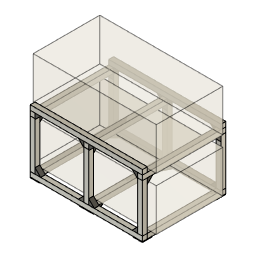
Battery Rack v4 (Autodesk Fusion 360 design; units mm, degrees)
Autodesk Fusion 360 part; units mm, degrees
note: some values were not read from the file. Chosen so that the rebuilt part matches the saved one: which bodies a step acts on.
sketch "Sketch1" plane through (0, 0, 0) normal (0, 0, 1) x (1, 0, 0)
  line L0 (-350, 260) -> (350, 260)
  line L1 (350, 260) -> (350, 230)
  line L2 (350, 230) -> (-350, 230)
  line L3 (-350, 230) -> (-350, 260)
  line L4 (-350, 230) -> (-320, 230)
  line L5 (-320, 230) -> (-320, -230)
  line L6 (-320, -230) -> (-350, -230)
  line L7 (-350, -230) -> (-350, 230)
  line L8 (-350, -230) -> (350, -230)
  line L9 (350, -230) -> (350, -260)
  line L10 (350, -260) -> (-350, -260)
  line L11 (-350, -260) -> (-350, -230)
  line L12 (350, -230) -> (320, -230)
  line L13 (320, -230) -> (320, 230)
  line L14 (320, 230) -> (350, 230)
  line L15 (350, 230) -> (350, -230)
  line L16 (0, 260) -> (0, -260) construction
  line L17 (-15, 230) -> (15, 230)
  line L18 (15, 230) -> (15, -230)
  line L19 (15, -230) -> (-15, -230)
  line L20 (-15, -230) -> (-15, 230)
  line L21 (350, 0) -> (-350, 0) construction
  line L22 (0, 1.75) -> (0, 22.5)
  line L23 (1.75, 0) -> (22.5, 0)
  dimension "d1" = 700
  dimension "d2" = 30
  dimension "d3" = 30
  dimension "d6" = 30
  dimension "d7" = 30
  dimension "d9" = 30
  dimension "d11" = 15
  dimension "d70" = 460
  constraint horizontal L0
  constraint vertical L1
  constraint horizontal L2
  constraint vertical L3
  constraint horizontal L4
  constraint vertical L5
  constraint horizontal L6
  constraint vertical L7
  constraint horizontal L8
  constraint vertical L9
  constraint horizontal L10
  constraint vertical L11
  constraint horizontal L12
  constraint vertical L13
  constraint horizontal L14
  constraint vertical L15
  constraint midpoint L0 L16.start
  constraint midpoint L10 L16.end
  constraint horizontal L17
  constraint vertical L18
  constraint horizontal L19
  constraint vertical L20
  constraint coincident L2 L17.start
  constraint midpoint L15 L21.start
  constraint midpoint L7 L21.end
  constraint collinear L16 L22
  constraint collinear L21 L23
  constraint collinear L8 L19
  measures "d1" distance of L0.start L0.end
  measures "d2" distance of L0.start L2.end
  measures "d3" distance of L2.end L4.end
  measures "d6" distance of L6.end L10.end
  measures "d7" distance of L8.end L12.end
  measures "d9" distance of L17.start L17.end
  measures "d11" distance of L16 L18
  measures "d70" distance of L4 L6
extrude "Extrude1" add sketch "Sketch1" along normal blind 30 contours L2 L4 L5 L6 L7 L8 makes body 1
extrude "Extrude2" add sketch "Sketch1" along normal blind 30 separate body contours L6 L8 L9 L10 L11 L12 L19 makes body 2
extrude "Extrude3" add sketch "Sketch1" along normal blind 30 separate body contours L2 L8 L17 L18 L19 L20 makes body 3
extrude "Extrude4" add sketch "Sketch1" along normal blind 30 separate body contours L0 L1 L2 L3 L4 L14 L17 makes body 4
extrude "Extrude5" add sketch "Sketch1" along normal blind 30 separate body contours L2 L8 L12 L13 L14 L15 makes body 5
sketch "Sketch2" plane through (0, 0, 0) normal (0, 0, 1) x (1, 0, 0)
  line L0 (350, -260) -> (-350, -260)
  line L1 (-350, -260) -> (-350, -230)
  line L2 (-350, -230) -> (-350, 230)
  circle A0 centre (-335, -245) radius 3
  circle A1 centre (-320, -245) radius 3
  circle A2 centre (-305, -245) radius 3
  circle A3 centre (-335, -230) radius 3
  circle A4 centre (-335, -215) radius 3
  line L3 (-350, -260) -> (-290, -260)
  line L4 (-290, -260) -> (-290, -200)
  line L5 (-290, -200) -> (-350, -200)
  line L6 (-350, -200) -> (-350, -260)
  line L7 (-290, -230) -> (-320, -200)
  dimension "d22" = 6
  dimension "d26" = 30
  dimension "d27" = 30
  dimension "d28" = 15
  dimension "d29" = 15
  dimension "d30" = 60
  dimension "d31" = 60
  dimension "d32" = 30
  dimension "d33" = 30
  constraint horizontal L3
  constraint vertical L4
  constraint horizontal L5
  constraint vertical L6
  constraint coincident L0.end L1.start
  constraint coincident L4 L7.start
  constraint coincident L5 L7.end
  measures "d22" diameter of A0
  measures "d28" distance of L0 A0.centre
  measures "d29" distance of L1 A0.centre
  measures "d30" distance of L0.end L3.end
  measures "d31" distance of L0.end L5.end
  measures "d32" distance of L5.end L7.end
  measures "d33" distance of L3.end L7.start
extrude "Extrude6" add sketch "Sketch2" against normal blind 4 separate body contours L0 L1 L2 L3 L4 L5 L6 L7 makes body 6
pattern_circular "C-Pattern1" count 2 over 360 about axis through (0, 0, 1.75) along (0, 0, 1) of bodies 6 makes body 7
mirror "Mirror1" about plane through (0, 0, 0) normal (0, 1, 0) of bodies 7 6 makes body 8 at (-305.2225, 224.0251, 0) makes body 9 at (305.2225, -224.0251, 0)
sketch "Sketch3" plane through (0, 0, 0) normal (0, 0, 1) x (1, 0, 0)
  circle A0 centre (-25, -245) radius 3
  line L0 (350, -260) -> (-350, -260)
  line L1 (0, 260) -> (0, -260)
  line L2 (-45, -260) -> (45, -260)
  line L3 (45, -260) -> (45, -170)
  line L4 (45, -170) -> (-45, -170)
  line L5 (-45, -170) -> (-45, -260)
  line L6 (45, -230) -> (15, -170)
  line L7 (-15, -170) -> (-45, -230)
  circle A1 centre (0, -245) radius 3
  circle A2 centre (25, -245) radius 3
  circle A3 centre (0, -220) radius 3
  circle A4 centre (0, -195) radius 3
  dimension "d40" = 6
  dimension "d43" = 50
  dimension "d44" = 50
  dimension "d47" = 90
  dimension "d48" = 90
  dimension "d49" = 45
  dimension "d51" = 30
  dimension "d52" = 30
  dimension "d53" = 30
  dimension "d54" = 30
  dimension "d115" = 15
  constraint horizontal L2
  constraint vertical L3
  constraint horizontal L4
  constraint vertical L5
  constraint coincident L0 L2.start
  constraint coincident L3 L6.start
  constraint coincident L4 L6.end
  constraint coincident L4 L7.start
  constraint coincident L5 L7.end
  constraint coincident L1 A1.centre
  measures "d40" diameter of A0
  measures "d47" distance of L2.start L2.end
  measures "d48" distance of L2.start L4.end
  measures "d49" distance of L1 L5
  measures "d51" distance of L2 L6.start
  measures "d52" distance of L2.start L7.end
  measures "d53" distance of L3.end L6.end
  measures "d54" distance of L4.end L7.start
  measures "d115" distance of L2 A1.centre
extrude "Extrude7" add sketch "Sketch3" against normal blind 4 separate body contours L0 L1 L2 L3 L4 L6 A1 A3 A4 | L0 L1 L2 L4 L5 L7 A1 A3 A4 makes body 10
mirror "Mirror2" about plane through (0, 0, 0) normal (0, 1, 0) of bodies 10 makes body 11
sketch "Sketch5" plane through (0, 0, 30) normal (0, 0, 1) x (-1, 0, 0)
  line L0 (15, 230) -> (-15, 230)
  line L1 (-15, 230) -> (-15, -230)
  line L2 (-15, -230) -> (15, -230)
  line L3 (15, -230) -> (15, 230)
  line L4 (383.75, -207.5) -> (-383.75, -207.5)
  line L5 (-383.75, -207.5) -> (-383.75, 207.5)
  line L6 (-383.75, 207.5) -> (383.75, 207.5)
  line L7 (383.75, 207.5) -> (383.75, -207.5)
  line L8 (-383.75, 0) -> (383.75, 0) construction
  line L9 (0, -207.5) -> (0, 207.5) construction
  line L10 (-1.75, 0) -> (-22.5, 0)
  dimension "d61" = 767.5
  dimension "d62" = 415
  dimension "d63" = 15
  constraint horizontal L4
  constraint vertical L5
  constraint horizontal L6
  constraint vertical L7
  constraint midpoint L5 L8.start
  constraint midpoint L7 L8.end
  constraint midpoint L4 L9.start
  constraint midpoint L6 L9.end
  constraint collinear L8 L10
  measures "d61" distance of L4.start L4.end
  measures "d62" distance of L4.start L6.end
  measures "d63" distance of L1 L9
extrude "Extrude9" add sketch "Sketch5" along normal blind 263 separate body contours L3 L4 L6 L7 | L1 L3 L4 L6 | L1 L4 L5 L6 makes body 12
sketch "Sketch4" plane through (0, 0, 30) normal (0, 0, 1) x (-1, 0, 0)
  line L0 (15, 230) -> (-15, 230)
  line L1 (-15, 230) -> (-15, -230)
  line L2 (-15, -230) -> (15, -230)
  line L3 (15, -230) -> (15, 230)
  line L4 (350, -230) -> (-350, -230)
  line L5 (-350, -230) -> (-350, -260)
  line L6 (-350, -260) -> (350, -260)
  line L7 (350, -260) -> (350, -230)
  line L8 (350, -230) -> (350, 230)
  line L9 (350, 230) -> (320, 230)
  line L10 (320, 230) -> (320, -230)
  line L11 (320, -230) -> (350, -230)
  line L12 (-350, 230) -> (350, 230)
  line L13 (350, 230) -> (350, 260)
  line L14 (350, 260) -> (-350, 260)
  line L15 (-350, 260) -> (-350, 230)
  line L16 (-350, -230) -> (-320, -230)
  line L17 (-320, -230) -> (-320, 230)
  line L18 (-320, 230) -> (-350, 230)
  line L19 (-350, 230) -> (-350, -230)
  line L20 (350, -260) -> (320, -260)
  line L21 (320, -260) -> (320, -230)
  line L22 (320, -230) -> (350, -230)
  line L23 (350, -230) -> (350, -260)
  line L24 (350, 230) -> (320, 230)
  line L25 (320, 230) -> (320, 260)
  line L26 (320, 260) -> (350, 260)
  line L27 (350, 260) -> (350, 230)
  line L28 (-320, 230) -> (-350, 230)
  line L29 (-350, 230) -> (-350, 260)
  line L30 (-350, 260) -> (-320, 260)
  line L31 (-320, 260) -> (-320, 230)
  line L32 (-320, -230) -> (-350, -230)
  line L33 (-350, -230) -> (-350, -260)
  line L34 (-350, -260) -> (-320, -260)
  line L35 (-320, -260) -> (-320, -230)
  line L36 (-15, -230) -> (15, -230)
  line L37 (15, -230) -> (15, -260)
  line L38 (15, -260) -> (-15, -260)
  line L39 (-15, -260) -> (-15, -230)
  line L40 (-15, 230) -> (15, 230)
  line L41 (15, 230) -> (15, 260)
  line L42 (15, 260) -> (-15, 260)
  line L43 (-15, 260) -> (-15, 230)
  constraint horizontal L20
  constraint vertical L21
  constraint horizontal L22
  constraint vertical L23
  constraint coincident L10.end L11.start
  constraint coincident L6.end L7.start
  constraint horizontal L24
  constraint vertical L25
  constraint horizontal L26
  constraint vertical L27
  constraint coincident L14 L25.end
  constraint coincident L8.end L9.start
  constraint horizontal L28
  constraint vertical L29
  constraint horizontal L30
  constraint vertical L31
  constraint coincident L14.end L15.start
  constraint coincident L17.end L18.start
  constraint horizontal L32
  constraint vertical L33
  constraint horizontal L34
  constraint vertical L35
  constraint coincident L5.end L6.start
  constraint coincident L16.end L17.start
  constraint horizontal L36
  constraint vertical L37
  constraint horizontal L38
  constraint vertical L39
  constraint coincident L6 L37.end
  constraint coincident L1.end L2.start
  constraint horizontal L40
  constraint vertical L41
  constraint horizontal L42
  constraint vertical L43
  constraint coincident L14 L41.end
  constraint coincident L0.end L1.start
  constraint collinear L10 L25
extrude "Extrude8" add sketch "Sketch4" along normal blind 300 separate body contours L0 L12 L14 L40 L41 L42 L43 | L2 L4 L6 L36 L37 L38 L39 | L9 L12 L13 L14 L24 L25 L26 L27 | L12 L14 L15 L18 L28 L29 L30 L31 | L4 L6 L7 L11 L20 L21 L22 L23 | L4 L5 L6 L16 L32 L33 L34 L35 makes body 13 at (340, -230, 130) makes body 14 at (-340, 230, 130) makes body 15 at (-5, -230, 130) makes body 16 at (340, 260, 130) makes body 17 at (5, 260, 130) makes body 18 at (-340, -260, 130)
pattern_linear "R-Pattern1" count 2 spacing 330 along (0, 0, 1) of bodies 1 5 3 makes body 19 at (-340, 76.6667, 330) makes body 20 at (-15, -76.6667, 340) makes body 21 at (340, 76.6667, 330)
pattern_linear "R-Pattern2" count 2 spacing 330 along (0, 0, 1) of bodies 12 makes body 22
move_face "OffsetFaces1" offset 30 3 faces at (340, 230, 340) (5, 230, 340) (-330, 230, 340) on bodies 19 20 21
move_face "OffsetFaces2" offset 30 3 faces at (330, -230, 340) (-5, -230, 340) (-330, -230, 350) on bodies 19 20 21
sketch "Sketch6" plane through (350, 0, 0) normal (1, 0, 0) x (0, 1, 0)
  line L0 (-260, 330) -> (260, 330)
  line L1 (260, 330) -> (260, 360)
  line L2 (260, 360) -> (-260, 360)
  line L3 (-260, 360) -> (-260, 330)
  line L4 (-230, 30) -> (-230, 330)
  line L5 (-230, 330) -> (-195, 330)
  line L6 (-195, 330) -> (-195, 295)
  line L7 (-195, 295) -> (-230, 295)
  line L8 (-230, 295) -> (-230, 330)
  line L9 (-195, 330) -> (-230, 295)
  dimension "d77" = 35
  dimension "d78" = 35
  constraint horizontal L5
  constraint vertical L6
  constraint horizontal L7
  constraint vertical L8
  constraint coincident L4.end L5.start
  measures "d77" distance of L4.end L5.end
  measures "d78" distance of L4.end L7.end
extrude "Extrude10" add sketch "Sketch6" against normal blind 30 separate body contours L0 L4 L5 L8 L9 makes body 23
pattern_linear "R-Pattern3" count 3 spacing 335 along (-1, 0, 0) of bodies 23 makes body 24 at (5, -206.6667, 318.3333) makes body 25 at (-330, -206.6667, 318.3333)
mirror "Mirror3" about plane through (0, 0, 0) normal (0, 1, 0) of bodies 23 24 25 makes body 26 at (340, 206.6667, 318.3333) makes body 27 at (5, 206.6667, 318.3333) makes body 28 at (-330, 206.6667, 318.3333)
sketch "Sketch7" plane through (0, -260, 0) normal (0, -1, 0) x (1, 0, 0)
  line L0 (-350, 0) -> (350, 0)
  line L1 (350, 0) -> (350, 30)
  line L2 (350, 30) -> (-350, 30)
  line L3 (-350, 30) -> (-350, 0)
  line L4 (320, 30) -> (320, 330)
  line L5 (320, 30) -> (285, 30)
  line L6 (285, 30) -> (285, 65)
  line L7 (285, 65) -> (320, 65)
  line L8 (320, 65) -> (320, 30)
  line L9 (320, 65) -> (285, 30)
  dimension "d87" = 35
  dimension "d88" = 35
  constraint horizontal L5
  constraint vertical L6
  constraint horizontal L7
  constraint vertical L8
  constraint coincident L4.start L5.start
  measures "d87" distance of L4.start L5.end
  measures "d88" distance of L4.start L7.end
extrude "Extrude11" add sketch "Sketch7" against normal blind 30 separate body contours L2 L4 L5 L8 L9 makes body 29
pattern_linear "R-Pattern4" count 2 spacing 335 along (-1, 0, 0) count 2 spacing 490 along (0, 1, 0) of bodies 29 makes body 30 at (-26.6667, -240, 53.3333) makes body 31 at (308.3333, 250, 53.3333) makes body 32 at (-26.6667, 250, 53.3333)
pattern_circular "C-Pattern2" count 2 over 360 about axis through (0, 0, 1.75) along (0, 0, 1) of bodies 29 30 31 32 makes body 33 at (-308.3333, 250, 53.3333) makes body 34 at (26.6667, 240, 53.3333) makes body 35 at (-308.3333, -250, 53.3333) makes body 36 at (26.6667, -250, 53.3333)
sketch "Sketch8" plane through (0, 260, 0) normal (0, 1, 0) x (-1, 0, 0)
  line L0 (-350, 330) -> (-320, 330)
  line L1 (-320, 330) -> (-320, 360)
  line L2 (-320, 360) -> (-350, 360)
  line L3 (-350, 360) -> (-350, 330)
  line L4 (320, 330) -> (350, 330)
  line L5 (350, 330) -> (350, 360)
  line L6 (350, 360) -> (320, 360)
  line L7 (320, 360) -> (320, 330)
  line L8 (-350, 360) -> (350, 360)
  line L9 (350, 360) -> (350, 390)
  line L10 (350, 390) -> (-350, 390)
  line L11 (-350, 390) -> (-350, 360)
  dimension "d97" = 30
  constraint horizontal L8
  constraint vertical L9
  constraint horizontal L10
  constraint vertical L11
  constraint coincident L2.end L3.start
  constraint collinear L5 L9
  measures "d97" distance of L2.end L10.end
extrude "Extrude12" add sketch "Sketch8" against normal blind 30 separate body contours L2 L6 L8 L9 L10 L11 makes body 37
sketch "Sketch9" plane through (0, 260, 0) normal (0, 1, 0) x (-1, 0, 0)
  line L0 (-350, 390) -> (-350, 360)
  line L1 (-350, 360) -> (350, 360)
  line L2 (350, 360) -> (350, 390)
  line L3 (350, 390) -> (-350, 390)
  line L4 (320, 330) -> (350, 330)
  line L5 (350, 330) -> (350, 360)
  line L6 (350, 360) -> (320, 360)
  line L7 (320, 360) -> (320, 330)
  line L8 (320, 360) -> (285, 360)
  line L9 (285, 360) -> (285, 325)
  line L10 (285, 325) -> (320, 325)
  line L11 (320, 325) -> (320, 360)
  line L12 (285, 360) -> (320, 325)
  dimension "d100" = 35
  dimension "d101" = 35
  constraint horizontal L8
  constraint vertical L9
  constraint horizontal L10
  constraint vertical L11
  constraint coincident L6.end L7.start
  measures "d100" distance of L6.end L8.end
  measures "d101" distance of L6.end L10.end
extrude "Extrude13" add sketch "Sketch9" against normal blind 30 separate body contours L1 L7 L8 L11 L12 makes body 38
pattern_linear "R-Pattern5" count 2 spacing 490 along (0, -1, 0) count 2 spacing 335 along (1, 0, 0) of bodies 38 makes body 39 at (-296.6667, -240, 348.3333) makes body 40 at (38.3333, 250, 348.3333) makes body 41 at (38.3333, -240, 348.3333)
pattern_circular "C-Pattern3" count 2 over 360 about axis through (0, 0, 1.75) along (0, 0, 1) of bodies 38 40 41 39 makes body 42 at (296.6667, -240, 348.3333) makes body 43 at (296.6667, 250, 348.3333) makes body 44 at (-38.3333, -250, 348.3333) makes body 45 at (-38.3333, 240, 348.3333)
pattern_linear "R-Pattern6" count 1 spacing 0 along (1, 0, 0) count 2 spacing 490 along (0, -1, 0) of bodies 37 makes body 46
named bodies: "Rack", "Rack (2)"
